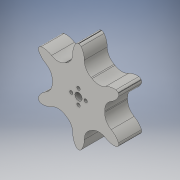
# Autodesk Inventor part: Pull Wheels
Saved by Autodesk Inventor 2016 (Build 200138000, 138)
## iProperties
Created: 2015-11-25
Part Number: Pull Wheels
Material: Generic
Document SubType Name: Modeling
Designer: luv2s
Density: 1 g/cm^3
Appearance: Default
Author: luv2s
Autodesk Inventor part; units mm, degrees
ref_plane "YZ Plane" through (0, 0, 0) normal (1, 0, 0) x (0, 1, 0)
ref_plane "XZ Plane" through (0, 0, 0) normal (0, 1, 0) x (-1, 0, 0)
ref_plane "XY Plane" through (0, 0, 0) normal (0, 0, 1) x (1, 0, 0)
sketch "Sketch1" plane through (0, 0, 0) normal (0, 0, 1) x (1, 0, 0)
  circle A0 centre (0, 0) radius 50.8
  line L0 (0, 50.8) -> (0, 25.4)
  line L1 (0, 25.4) -> (13.97, 25.4)
  line L2 (0, 38.1) -> (6.35, 38.1)
  arc A1 (6.35, 38.1) -> (13.97, 25.4) centre (20.3177, 37.8446) ccw
  line L3 (35.921, 35.921) -> (0, 0)
  line L4 (0, 50.8) -> (0, 0)
  arc A2 (1.9047, 50.7643) -> (0, 50.8) centre (-0.9526, -50.7955) ccw
  arc A3 (6.35, 38.1) -> (1.9047, 50.7643) centre (-12.909, 38.4522) ccw
  line L5 (0, 25.4) -> (-13.97, 25.4)
  arc A4 (-13.97, 25.4) -> (-6.35, 38.1) centre (-20.3177, 37.8446) ccw
  arc A5 (0, 50.8) -> (-1.9047, 50.7643) centre (0.9526, -50.7955) ccw
  arc A6 (-1.9047, 50.7643) -> (-6.35, 38.1) centre (12.909, 38.4522) ccw
  arc A7 (-29.8206, 24.5493) -> (-43.0108, 27.0316) centre (-39.755, 8.0465) ccw
  arc A8 (-43.9941, 25.4) -> (-44.9155, 23.7327) centre (44.4665, -24.5728) ccw
  arc A9 (-43.0108, 27.0316) -> (-43.9941, 25.4) centre (43.5139, -26.2227) ccw
  arc A10 (-44.9155, 23.7327) -> (-36.1706, 13.5507) centre (-26.846, 30.4056) ccw
  arc A11 (-28.982, 0.6016) -> (-36.1706, 13.5507) centre (-42.9332, 1.3267) ccw
  arc A12 (-29.8206, 24.5493) -> (-15.012, 24.7984) centre (-22.6156, 36.5179) ccw
  arc A13 (-36.1706, -13.5507) -> (-44.9155, -23.7327) centre (-26.846, -30.4056) ccw
  arc A14 (-43.9941, -25.4) -> (-43.0108, -27.0316) centre (43.5139, 26.2227) ccw
  arc A15 (-44.9155, -23.7327) -> (-43.9941, -25.4) centre (44.4665, 24.5728) ccw
  arc A16 (-43.0108, -27.0316) -> (-29.8206, -24.5493) centre (-39.755, -8.0465) ccw
  arc A17 (-15.012, -24.7984) -> (-29.8206, -24.5493) centre (-22.6156, -36.5179) ccw
  arc A18 (-36.1706, -13.5507) -> (-28.982, -0.6016) centre (-42.9332, -1.3267) ccw
  arc A19 (-6.35, -38.1) -> (-1.9047, -50.7643) centre (12.909, -38.4522) ccw
  arc A20 (0, -50.8) -> (1.9047, -50.7643) centre (-0.9526, 50.7955) ccw
  arc A21 (-1.9047, -50.7643) -> (0, -50.8) centre (0.9526, 50.7955) ccw
  arc A22 (1.9047, -50.7643) -> (6.35, -38.1) centre (-12.909, -38.4522) ccw
  arc A23 (13.97, -25.4) -> (6.35, -38.1) centre (20.3177, -37.8446) ccw
  arc A24 (-6.35, -38.1) -> (-13.97, -25.4) centre (-20.3177, -37.8446) ccw
  arc A25 (29.8206, -24.5493) -> (43.0108, -27.0316) centre (39.755, -8.0465) ccw
  arc A26 (43.9941, -25.4) -> (44.9155, -23.7327) centre (-44.4665, 24.5728) ccw
  arc A27 (43.0108, -27.0316) -> (43.9941, -25.4) centre (-43.5139, 26.2227) ccw
  arc A28 (44.9155, -23.7327) -> (36.1706, -13.5507) centre (26.846, -30.4056) ccw
  arc A29 (28.982, -0.6016) -> (36.1706, -13.5507) centre (42.9332, -1.3267) ccw
  arc A30 (29.8206, -24.5493) -> (15.012, -24.7984) centre (22.6156, -36.5179) ccw
  arc A31 (36.1706, 13.5507) -> (44.9155, 23.7327) centre (26.846, 30.4056) ccw
  arc A32 (43.9941, 25.4) -> (43.0108, 27.0316) centre (-43.5139, -26.2227) ccw
  arc A33 (44.9155, 23.7327) -> (43.9941, 25.4) centre (-44.4665, -24.5728) ccw
  arc A34 (43.0108, 27.0316) -> (29.8206, 24.5493) centre (39.755, 8.0465) ccw
  arc A35 (15.012, 24.7984) -> (29.8206, 24.5493) centre (22.6156, 36.5179) ccw
  arc A36 (36.1706, 13.5507) -> (28.982, 0.6016) centre (42.9332, 1.3267) ccw
  line L6 (-28.982, -0.6016) -> (-28.982, 0.6016)
  line L7 (28.982, -0.6016) -> (28.982, 0.6016)
  line L8 (15.012, 24.7984) -> (13.97, 25.4)
  line L9 (-15.012, 24.7984) -> (-13.97, 25.4)
  line L10 (-15.012, -24.7984) -> (-13.97, -25.4)
  line L11 (13.97, -25.4) -> (15.012, -24.7984)
  dimension "d0" = 101.6
  dimension "d1" = 25.4
  dimension "d2" = 13.97
  dimension "d7" = 45
  dimension "d8" = 13.97
  dimension "d10" = 6.35
  dimension "d11" = 1.905
  dimension "d15" = 360
  constraints: 76 point on circle, 37 centre point, 24 end point, 6 symmetric about line, 3 parallel, 2 vertical, 1 coincident, 1 collinear, 1 horizontal, 1 midpoint, 1 perpendicular, 1 tangent, 118 other
  measures "d0" diameter of A0
  measures "d1" distance of L0.start L0.end
  measures "d2" distance of L0.end L1.end
  measures "d7" angle of L3 L4
  measures "d8" radius of A1
  measures "d10" distance of L2.start L2.end
  measures "d11" distance of L0.start A2.start
extrude "Extrusion1" add sketch "Sketch1" along normal blind 25.4 contours A31 A36 L7 A29 A28 A26 A27 A25 A30 L11 A23 A22 A20 A21 A19 A24 L10 A17 A16 A14 A15 A13 A18 L6 A11 A10 A8 A9 A7 A12 L9 L5 L4 L3 A35 A34 A32 A33 | L3 L4 L1 L8 A35 | L0 L5 A4 A6 A5 | A1 L1 L0 L2
extrude "Extrusion2" add sketch "Sketch1" along normal blind 25.4 contours A3 L2 L0 A2
fillet "Fillet1" radius 3.175 18 edges at (44.9155, 23.7327, 12.7) (43.0108, 27.0316, 12.7) (1.9047, 50.7643, 12.7) (-1.9047, 50.7643, 12.7) (0, 50.8, 12.7) (43.9941, 25.4, 12.7) (44.9155, -23.7327, 12.7) (43.9941, -25.4, 12.7) (43.0108, -27.0316, 12.7) (1.9047, -50.7643, 12.7) (-1.9047, -50.7643, 12.7) (0, -50.8, 12.7) (-43.0108, -27.0316, 12.7) (-43.9941, -25.4, 12.7) (-44.9155, -23.7327, 12.7) (-44.9155, 23.7327, 12.7) (-43.9941, 25.4, 12.7) (-43.0108, 27.0316, 12.7)
sketch "Sketch2" plane through (0, 0, 0) normal (0, 0, -1) x (-1, 0, 0)
  line L0 (0, 0) -> (-8, 0)
  line L1 (0, 0) -> (8, 0)
  circle A0 centre (-8, 0) radius 1.8542
  circle A1 centre (8, 0) radius 1.8542
  line L2 (0, 0) -> (0, -8.001)
  line L3 (0, -8.001) -> (0, 8.001)
  circle A2 centre (0, 8.001) radius 1.8542
  circle A3 centre (0, -8.001) radius 1.85
  circle A4 centre (0, 0) radius 4
  dimension "d22" = 8
  dimension "d23" = 8
  dimension "d24" = 3.7084
  dimension "d25" = 3.7084
  dimension "d26" = 8.001
  dimension "d27" = 16.002
  dimension "d28" = 3.7084
  dimension "d29" = 3.7
  dimension "d30" = 8
  constraints: 8 end point, 5 centre point, 5 coincident, 2 horizontal, 1 point on line, 1 vertical
  measures "d22" distance of L0.start L0.end
  measures "d23" distance of L0.start L1.end
  measures "d24" diameter of A0
  measures "d25" diameter of A1
  measures "d26" distance of L0.start L2.end
  measures "d27" distance of L2.end L3.end
  measures "d28" diameter of A2
  measures "d29" diameter of A3
  measures "d30" diameter of A4
extrude "Extrusion3" cut sketch "Sketch2" against normal blind 25.4
body "Solid1"
